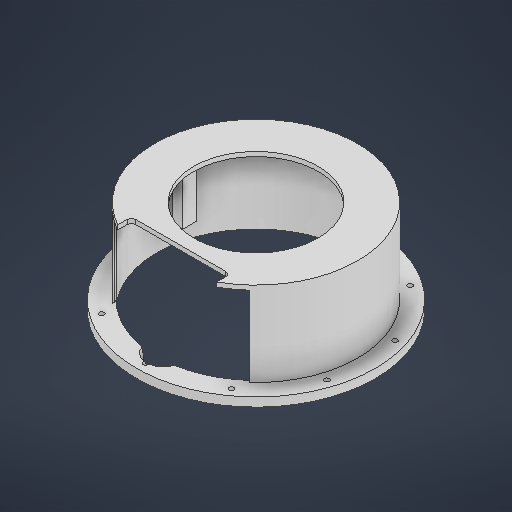
# Autodesk Inventor part: Cylinder Segment  Camera only
Saved by Autodesk Inventor 2025 (Build 290162000, 162)
## iProperties
Created: 2024-04-11
Part Number: Cylinder Segment  Camera only
Material: Generic
Document SubType Name: Modeling
Designer: Thienan Hoang
Density: 1 g/cm^3
Appearance: Default
Author: Thienan Hoang
Autodesk Inventor part; units mm, degrees
ref_plane "YZ Plane" through (0, 0, 0) normal (1, 0, 0) x (0, 1, 0)
ref_plane "XZ Plane" through (0, 0, 0) normal (0, 1, 0) x (-1, 0, 0)
ref_plane "XY Plane" through (0, 0, 0) normal (0, 0, 1) x (1, 0, 0)
sketch "Sketch1" plane through (0, 0, 0) normal (0, 1, 0) x (-1, 0, 0)
  circle A0 centre (0, 0) radius 135
  circle A1 centre (0, 0) radius 115
  circle A2 centre (0, 0) radius 112.0375
  circle A3 centre (0, 0) radius 9.5
  circle A4 centre (0, 0) radius 125
  circle A5 centre (0, -125) radius 2.75
  circle A6 centre (73.4732, -101.1271) radius 2.75
  circle A7 centre (118.8821, -38.6271) radius 2.75
  circle A8 centre (118.8821, 38.6271) radius 2.75
  circle A9 centre (73.4732, 101.1271) radius 2.75
  circle A10 centre (0, 125) radius 2.75
  circle A11 centre (-73.4732, 101.1271) radius 2.75
  circle A12 centre (-118.8821, 38.6271) radius 2.75
  circle A13 centre (-118.8821, -38.6271) radius 2.75
  circle A14 centre (-73.4732, -101.1271) radius 2.75
  dimension "d264" = 250
  dimension "Absolute_Diameter" = 270
  dimension "Diameter_No_Outer_Lip" = 230
  dimension "Inner_Cylinder_Diameter" = 224.075
  dimension "Lip_Diameter" = 19
  dimension "d265" = 5.5
  dimension "d268" = 360
  constraints: 14 centre point, 5 coincident, 1 vertical alignment, 23 other
  measures "Absolute_Diameter" diameter of A0
  measures "Diameter_No_Outer_Lip" diameter of A1
  measures "Inner_Cylinder_Diameter" diameter of A2
  measures "Lip_Diameter" diameter of A3
  measures "d265" diameter of A5
extrude "Extrusion1" add sketch "Sketch1" along normal blind 10 contours A0 | A4 A7 A6 A5 A14 A13 A12 A11 A10 A9 A8
extrude "Extrusion2" add sketch "Sketch1" along normal blind 105.5 contours A1
sketch "Sketch2" plane through (0, 105.5, 0) normal (0, 1, 0) x (1, 0, 0)
  circle A0 centre (0, 0) radius 115
  circle A1 centre (0, 0) radius 70.375
  dimension "Lip_Diameter_Out" = 230
  dimension "Inner_Lip_Diameter" = 140.75
  constraints: 2 centre point, 1 coincident
  measures "Lip_Diameter_Out" diameter of A0
  measures "Inner_Lip_Diameter" diameter of A1
extrude "Extrusion7" add sketch "Sketch2" against normal blind 5
sketch "Sketch28" plane through (0, 10, 0) normal (0, 1, 0) x (1, 0, 0)
  line L0 (-77.5, -75) -> (77.5, -75)
  line L1 (77.5, -75) -> (77.5, -175)
  line L2 (77.5, -175) -> (-77.5, -175)
  line L3 (-77.5, -175) -> (-77.5, -75)
  circle A0 centre (0, -125) radius 2.75 projected
  line L4 (-77.5, -75) -> (77.5, -175) construction
  line L5 (77.5, -75) -> (-77.5, -175) construction
  point P0 (0, 0)
  dimension "d271" = 155
  dimension "d272" = 100
  constraints: 12 end point, 2 midpoint, 2 parallel, 1 horizontal, 1 perpendicular
  measures "d271" distance of L1.end L2.end
  measures "d272" distance of L0.end L1.end
extrude "Extrusion34" cut sketch "Sketch28" along normal up to surface (90.5 mm away)
sketch "Sketch30" plane through (0, 10, 0) normal (0, 1, 0) x (1, 0, 0)
  point P0 (0, 0)
ref_plane "Work Plane19" through (16.25, 10, -160.125) normal (0, 0.3947439, -0.9187912) x (1, 0, 0)
ref_plane "Work Plane21" through (16.25, 10, -160.125) normal (0, 0.911762, 0.4107189) x (1, 0, 0)
ref_plane "Work Plane22" through (16.25, 101.1762, -119.0531) normal (0, 0.911762, 0.4107189) x (1, 0, 0)
sketch "Sketch31" plane through (16.25, 101.1762, -119.0531) normal (0, 0.911762, 0.4107189) x (1, 0, 0)
  circle A0 centre (-16.25, -239.1031) radius 20
  point P0 (-16.25, -150.1031)
  dimension "d286" = 40
  dimension "d289" = 89
  constraints: 1 centre point
  measures "d286" diameter of A0
  measures "d289" distance of point (-16.25, -150.103) A0.centre
extrude "Extrusion36" cut sketch "Sketch31" along normal mid plane 52.8625
fillet "Fillet19" radius 5 2 edges at (-77.5, 55.25, 80.9083) (77.5, 55.25, 80.9083)
sketch "Sketch32" plane through (0, 105.5, 0) normal (0, 1, 0) x (1, 0, 0)
  line L0 (-51, -85) -> (51, -85)
  line L1 (56, -90) -> (56, -125)
  line L2 (56, -125) -> (-56, -125)
  line L3 (-56, -125) -> (-56, -90)
  line L4 (-56, -85) -> (56, -125) construction
  line L5 (56, -85) -> (-56, -125) construction
  arc A0 (-51, -85) -> (-56, -90) centre (-51, -90) ccw
  arc A1 (56, -90) -> (51, -85) centre (51, -90) ccw
  point P0 (0, 0)
  point P1 (0, -105)
  point P2 (0, -85)
  dimension "d291" = 112
  dimension "d292" = 40
  dimension "d293" = 5
  dimension "d294" = 5
  dimension "d295" = 85
  constraints: 12 end point, 4 point on circle, 4 point on line, 4 tangent, 3 midpoint, 2 centre point, 2 parallel, 1 horizontal, 1 perpendicular
  measures "d291" distance of L1.end L2.end
  measures "d292" distance of L5.start L1.end
  measures "d293" radius of A0
  measures "d294" radius of A1
  measures "d295" distance of point (0, 0) point (0, -85)
extrude "Extrusion37" cut sketch "Sketch32" against normal blind 10
sketch "Sketch33" plane through (0, 100.5, 0) normal (0, -1, 0) x (1, 0, 0)
  circle A0 centre (0, 0) radius 68.375
  line L0 (-86.7392, 8) -> (-75, 8)
  line L1 (-75, 8) -> (-75, -8)
  line L2 (-75, -8) -> (-86.7392, -8)
  line L3 (-86.7392, -8) -> (-86.7392, 8)
  line L4 (-86.7392, 8) -> (-75, -8) construction
  line L5 (-75, 8) -> (-86.7392, -8) construction
  line L6 (0, 0) -> (0, 68.375)
  line L7 (86.7392, 8) -> (75, 8)
  line L8 (75, 8) -> (75, -8)
  line L9 (75, -8) -> (86.7392, -8)
  line L10 (86.7392, -8) -> (86.7392, 8)
  line L11 (86.7392, 8) -> (75, -8) construction
  line L12 (75, 8) -> (86.7392, -8) construction
  point P0 (-80.8696, 0)
  point P1 (80.8696, 0)
  point P2 (-75, 0)
  dimension "d298" = 16
  dimension "d301" = 75
  constraints: 26 end point, 5 symmetric about line, 3 midpoint, 2 parallel, 1 coincident, 1 horizontal, 1 perpendicular, 1 vertical, 1 vertical alignment, 2 other
  measures "d298" distance of L0.end L1.end
  measures "d301" distance of point (0, 0) point (-75, 0)
extrude "Extrusion38" add sketch "Sketch33" along normal blind 55 contours L0 L1 L2 L3 | L10 L9 L8 L7
sketch "Sketch35" plane through (0, 45.5, 0) normal (0, -1, 0) x (1, 0, 0)
  line L0 (0, 0) -> (0, 42.8625)
  circle A0 centre (0, 0) radius 81
  circle A1 centre (-81, 0) radius 3.25
  circle A2 centre (81, 0) radius 3.25
  circle A3 centre (0, 0) radius 87.5
  dimension "d308" = 162
  dimension "d309" = 6.5
  dimension "d312" = 175
  constraints: 3 centre point, 2 coincident, 2 end point, 1 horizontal alignment, 1 symmetric about line, 1 vertical, 3 other
  measures "d309" diameter of A1
  measures "d312" diameter of A3
extrude "Extrusion40" cut sketch "Sketch35" against normal blind 15 contours A0 A2 | A0 A2 | A1 A0 | A0 A1
body "Solid1"
